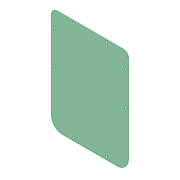
# Autodesk Inventor part: beagle_spacer_top
Saved by Autodesk Inventor 2014 (Build 180170000, 170)
## iProperties
Created: 2013-06-20
Part Number: beagle_spacer_top
Document SubType Name: Modeling
Designer: Administrator
Density: 1 g/cm^3
Material: Generic
Appearance: Clear - Green 1
Author: Administrator
Autodesk Inventor part; units mm, degrees
ref_plane "YZ Plane" through (0, 0, 0) normal (1, 0, 0) x (0, 1, 0)
ref_plane "XZ Plane" through (0, 0, 0) normal (0, 1, 0) x (-1, 0, 0)
ref_plane "XY Plane" through (0, 0, 0) normal (0, 0, 1) x (1, 0, 0)
sketch "Sketch1" plane through (0, 0, 0) normal (0, 0, 1) x (1, 0, 0)
  line L0 (9.8795, 48.1994) -> (9.8795, -53.4006)
  line L1 (16.2295, 54.5494) -> (92.4295, 54.5494)
  line L2 (98.7795, 48.1994) -> (98.7795, -53.4006)
  line L3 (22.5795, -66.1006) -> (86.0795, -66.1006)
  arc A0 (9.8795, -53.4006) -> (22.5795, -66.1006) centre (22.5795, -53.4006) ccw
  arc A1 (16.2295, 54.5494) -> (9.8795, 48.1994) centre (16.2295, 48.1994) ccw
  arc A2 (98.7795, 48.1994) -> (92.4295, 54.5494) centre (92.4295, 48.1994) ccw
  arc A3 (86.0795, -66.1006) -> (98.7795, -53.4006) centre (86.0795, -53.4006) ccw
  point P0 (0, 0)
  dimension "d0" = 12.7
  dimension "d1" = 6.35
  dimension "d2" = 120.65
  dimension "d3" = 88.9
  constraints: 8 end point, 8 point on circle, 8 tangent, 4 centre point, 2 equal radius, 1 horizontal, 1 vertical
  measures "d0" radius of A0
  measures "d1" radius of A1
  measures "d2" distance between parallel lines of L3 L1
  measures "d3" distance between parallel lines of L2 L0
extrude "Extrusion1" add sketch "Sketch1" along normal blind 0.7937
sketch "Sketch11" plane through (0, 0, 0.7937) normal (0, 0, 1) x (1, 0, 0)
  line L0 (9.8795, -53.4006) -> (9.8795, 48.1994) projected
  line L1 (86.0795, -66.1006) -> (22.5795, -66.1006) projected
  line L2 (98.7795, 48.1994) -> (98.7795, -53.4006) projected
  line L3 (16.2295, 54.5494) -> (92.4295, 54.5494) projected
  circle A0 centre (35.2795, 51.4252) radius 1.27
  circle A1 centre (73.3795, 51.4252) radius 1.27
  circle A2 centre (13.0037, 35.4994) radius 1.27
  circle A3 centre (13.0037, -2.6006) radius 1.27
  circle A4 centre (35.2795, -62.9764) radius 1.27
  circle A5 centre (73.3795, -62.9764) radius 1.27
  circle A6 centre (95.6553, 35.4994) radius 1.27
  circle A7 centre (95.6553, -2.6006) radius 1.27
  point P0 (0, 0)
  dimension "d122" = 3.1242
  dimension "d123" = 3.1242
  dimension "d124" = 3.1242
  dimension "d125" = 3.1242
  dimension "d126" = 25.4
  dimension "d127" = 38.1
  dimension "d128" = 19.05
  dimension "d129" = 38.1
  dimension "d130" = 2.54
  constraints: 8 centre point, 7 equal radius, 4 horizontal alignment, 4 vertical alignment
  measures "d122" distance from line of L3 A0.centre
  measures "d123" distance from line of L0 A2.centre
  measures "d124" distance from line of L2 A6.centre
  measures "d125" distance from line of L1 A4.centre
  measures "d126" distance from line of L0 A0.centre
  measures "d127" distance of A1.centre A0.centre
  measures "d128" distance from line of L3 A2.centre
  measures "d129" distance of A3.centre A2.centre
  measures "d130" diameter of A0
extrude "Extrusion19" cut sketch "Sketch11" against normal through all
body "Solid1"
